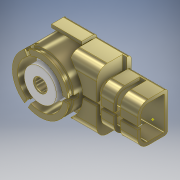
# Autodesk Inventor part: U.FL_Female
Saved by Autodesk Inventor 2018 (Build 220112000, 112)
## iProperties
Created: 2018-07-13
Part Number: U.FL_Female
Material: Copper
Document SubType Name: Modeling
Designer: Bradley
Density: 8.94 g/cm^3
Appearance: Gold - Metal
Author: Bradley
Autodesk Inventor part; units mm, degrees
ref_plane "YZ Plane" through (0, 0, 0) normal (1, 0, 0) x (0, 1, 0)
ref_plane "XZ Plane" through (0, 0, 0) normal (0, 1, 0) x (-1, 0, 0)
ref_plane "XY Plane" through (0, 0, 0) normal (0, 0, 1) x (1, 0, 0)
sketch "Sketch1" plane through (0, 0, 0) normal (0, 0, 1) x (1, 0, 0)
  line L0 (0, 0.565) -> (0, -0.565)
  line L1 (0, -0.565) -> (0.275, -0.565)
  line L2 (0.275, -0.565) -> (0.275, -1.365)
  line L3 (0.275, -1.365) -> (0.75, -1.365)
  line L4 (0.75, -1.365) -> (0.75, -0.495)
  line L5 (0.75, -0.495) -> (1.05, -0.495)
  line L6 (1.05, -0.495) -> (1.05, -1.365)
  line L7 (1.05, -1.365) -> (1.3, -1.365)
  line L8 (1.3, -1.365) -> (1.3, -1.295)
  line L9 (1.3, -1.295) -> (1.2, -1.295)
  line L10 (1.2, -1.295) -> (1.2, -1.095)
  line L11 (1.2, -1.095) -> (1.3, -1.095)
  line L12 (1.3, -1.095) -> (1.3, 0.565)
  line L13 (1.3, 0.565) -> (0, 0.565)
  point P0 (0, 0)
  point P1 (0, 0)
  dimension "d0" = 2.6
  dimension "d1" = 1.93
  dimension "d2" = 2.1
  dimension "d3" = 1.5
  dimension "d4" = 0.55
  dimension "d5" = 0.8
  dimension "d6" = 0.07
  dimension "d7" = 0.6
  dimension "d8" = 0.2
  dimension "d9" = 0.1
  constraints: 28 end point, 10 perpendicular, 4 point on line, 1 coincident, 1 midpoint, 1 vertical
  measures "d0" diameter of L12 L0
  measures "d1" distance between parallel lines of L7 L13
  measures "d2" diameter of L6 L0
  measures "d3" diameter of L4 L0
  measures "d4" diameter of L2 L0
  measures "d5" distance of L1.end L2.end
  measures "d6" distance between parallel lines of L5 L1
  measures "d7" distance between parallel lines of L11 L5
  measures "d8" distance of L9.end L10.end
  measures "d9" distance of L10.end L11.end
revolve "Revolution1" add sketch "Sketch1" angle 360 about axis through (0, 0.565, 0) along (0, -1, 0)
sketch "Sketch2" plane through (0, 0.565, 0) normal (0, 1, 0) x (1, 0, 0)
  circle A0 centre (0, 0) radius 1.3 projected
  line L0 (-0.7, -1.5) -> (0.7, -1.5)
  line L1 (0.7, -1.5) -> (0.7, 1.5)
  line L2 (0.7, 1.5) -> (-0.7, 1.5)
  line L3 (-0.7, 1.5) -> (-0.7, -1.5)
  line L4 (0.7, -1.25) -> (0.8, -1.25)
  line L5 (0.8, -1.25) -> (0.8, 1.25)
  line L6 (0.8, 1.25) -> (0.7, 1.25)
  line L7 (0.7, 1.25) -> (0.7, -1.25)
  point P0 (0, 0)
  point P1 (0, -1.5)
  point P2 (-0.7, 0)
  point P3 (0.7, 0)
  dimension "d11" = 1.4
  dimension "d12" = 3
  dimension "d13" = 2.5
  dimension "d14" = 0.1
  constraints: 16 end point, 4 midpoint, 4 parallel, 2 horizontal, 2 perpendicular, 1 horizontal alignment, 1 point on line, 1 vertical alignment
  measures "d11" distance of L0.start L0.end
  measures "d12" distance of L2.end L0.start
  measures "d13" distance of L4.end L5.end
  measures "d14" distance of L4.start L4.end
extrude "Extrusion1" add sketch "Sketch2" against normal blind 0.7 contours L5 A0 L1 | A0 L1 L6 L5 | L5 L4 L1 A0 | L1 A0 L3 | A0 L3 L2 L1 | L1 L0 L3 A0
sketch "Sketch3" plane through (-0.7, 0.565, -1.5) normal (0, 1, 0) x (1, 0, 0)
  arc A0 (1.5, -2.5247) -> (1.5, -0.4753) centre (0.7, -1.5) ccw projected
  line L0 (1.5, -0.4753) -> (1.5, -0.25) projected
  line L1 (1.5, -0.25) -> (1.4, -0.25) projected
  line L2 (1.4, -0.25) -> (1.4, 0) projected
  line L3 (1.4, 0) -> (0, 0) projected
  line L4 (0, 0) -> (0, -0.4046) projected
  arc A1 (0, -0.4046) -> (0, -2.5954) centre (0.7, -1.5) ccw projected
  line L5 (0, -2.5954) -> (0, -3) projected
  line L6 (0, -3) -> (1.4, -3) projected
  line L7 (1.4, -3) -> (1.4, -2.75) projected
  line L8 (1.4, -2.75) -> (1.5, -2.75) projected
  line L9 (1.5, -2.75) -> (1.5, -2.5247) projected
  line L10 (1.5, -0.075) -> (3, -0.075)
  line L11 (3, -0.075) -> (3, -2.925)
  line L12 (3, -2.925) -> (1.5, -2.925)
  line L13 (1.5, -2.925) -> (1.5, -0.075)
  line L14 (3, -0.575) -> (4.7, -0.575)
  line L15 (4.7, -0.575) -> (4.7, -2.425)
  line L16 (4.7, -2.425) -> (3, -2.425)
  line L17 (3, -2.425) -> (3, -0.575)
  arc A2 (1.5, -2.5247) -> (1.5, -0.4753) centre (0.7, -1.5) ccw
  arc A3 (1.5, -2.5247) -> (1.5, -0.4753) centre (0.7, -1.5) ccw projected
  point P0 (0.7, -1.5)
  point P1 (1.5, -1.5)
  point P2 (3, -1.5)
  dimension "d17" = 2.85
  dimension "d18" = 1.5
  dimension "d19" = 1.85
  dimension "d20" = 4
  constraints: 16 end point, 4 parallel, 4 point on circle, 3 midpoint, 3 point on line, 2 horizontal, 2 perpendicular, 1 centre point, 1 collinear, 1 concentric, 1 horizontal alignment
  measures "d17" distance of L10.end L11.end
  measures "d18" distance of L10.start L10.end
  measures "d19" distance of L14.end L15.end
  measures "d20" distance from line of L15 point (0.7, -1.5)
extrude "Extrusion2" add sketch "Sketch3" against normal blind 1.4 contours A0 L0 L13 L10 L11 L12 L9 | L11 L14 L15 L16
sketch "Sketch4" plane through (0, -1.365, 0) normal (0, -1, 0) x (1, 0, 0)
  circle A0 centre (0, 0) radius 1.3 projected
  circle A1 centre (0, 0) radius 1.05 projected
  circle A2 centre (0, 0) radius 1.05 projected
  arc A3 (1.0452, -0.1) -> (1.0452, 0.1) centre (0, 0) ccw
  circle A4 centre (0, 0) radius 1.3 projected
  arc A5 (1.2961, -0.1) -> (1.2961, 0.1) centre (0, 0) ccw
  line L0 (1.0452, 0.1) -> (1.2961, 0.1)
  line L1 (1.2961, -0.1) -> (1.0452, -0.1)
  circle A6 centre (0, 0) radius 1.05 projected
  arc A7 (-0.436, 0.9552) -> (-0.6092, 0.8552) centre (0, 0) ccw
  arc A8 (-0.5615, 1.1725) -> (-0.7347, 1.0725) centre (0, 0) ccw
  line L2 (-0.6092, 0.8552) -> (-0.7347, 1.0725)
  line L3 (-0.5615, 1.1725) -> (-0.436, 0.9552)
  arc A9 (-0.6092, -0.8552) -> (-0.436, -0.9552) centre (0, 0) ccw
  arc A10 (-0.7347, -1.0725) -> (-0.5615, -1.1725) centre (0, 0) ccw
  line L4 (-0.436, -0.9552) -> (-0.5615, -1.1725)
  line L5 (-0.7347, -1.0725) -> (-0.6092, -0.8552)
  point P0 (0, 0)
  dimension "d23" = 0.2
  dimension "d26" = 360
  constraints: 16 point on circle, 12 end point, 6 centre point, 2 concentric, 2 horizontal, 1 parallel, 31 other
  measures "d23" distance between parallel lines of L1 L0
extrude "Extrusion3" cut sketch "Sketch4" against normal blind 0.5 contours A0 L1 A1 L0 | L3 A1 L2 A0 | A0 L5 A1 L4
fillet "Fillet1" radius 0.5 4 edges at (1.55, -0.835, 1.425) (3.15, -0.835, 0.925) (1.55, -0.835, -1.425) (3.15, -0.835, -0.925)
sketch "Sketch5" plane through (1.0452, -1.365, -0.1) normal (0, -1, 0) x (1, 0, 0)
  arc A0 (-1.7452, -0.9954) -> (-0.2452, -0.9247) centre (-1.0452, 0.1) ccw projected
  line L0 (-1.7452, -0.9954) -> (-1.7452, -1.4) projected
  line L1 (-1.7452, -1.4) -> (-0.3452, -1.4) projected
  line L2 (-0.3452, -1.4) -> (-0.3452, -1.15) projected
  line L3 (-0.3452, -1.15) -> (-0.2452, -1.15) projected
  line L4 (-0.2452, -1.15) -> (-0.2452, -0.9247) projected
  arc A1 (-0.2452, 1.1247) -> (-1.7452, 1.1954) centre (-1.0452, 0.1) ccw projected
  line L5 (-0.2452, 1.1247) -> (-0.2452, 1.35) projected
  line L6 (-0.2452, 1.35) -> (-0.3452, 1.35) projected
  line L7 (-0.3452, 1.35) -> (-0.3452, 1.6) projected
  line L8 (-0.3452, 1.6) -> (-1.7452, 1.6) projected
  line L9 (-1.7452, 1.6) -> (-1.7452, 1.1954) projected
  line L10 (-1.7452, -0.9954) -> (-1.7452, -1.4) projected
  line L11 (-1.7452, -1.25) -> (-0.3452, -1.25)
  line L12 (-1.7452, 1.1954) -> (-1.7452, 1.6) projected
  line L13 (-1.7452, 1.45) -> (-0.3452, 1.45)
  line L14 (-0.3452, 1.6) -> (-0.3452, 1.35) projected
  line L15 (-0.2452, -0.9247) -> (-0.2452, -1.325) projected
  line L16 (-0.2452, -1.325) -> (1.2548, -1.325) projected
  line L17 (1.2548, -1.325) -> (1.2548, -0.825) projected
  line L18 (1.2548, -0.825) -> (-0.1318, -0.825) projected
  line L19 (2.9548, -0.325) -> (1.2548, -0.325) projected
  line L20 (2.9548, -0.325) -> (2.9548, 0.525) projected
  line L21 (1.2548, 0.525) -> (2.9548, 0.525) projected
  line L22 (1.2548, 1.025) -> (1.2548, 0.525) projected
  line L23 (-0.1318, 1.025) -> (1.2548, 1.025) projected
  arc A2 (-0.1318, -0.825) -> (-0.1318, 1.025) centre (-1.0452, 0.1) ccw projected
  line L24 (1.2548, -0.825) -> (-0.1318, -0.825) projected
  line L25 (1.2548, -0.325) -> (1.2548, -0.825) projected
  line L26 (-0.2452, 1.525) -> (-0.2452, 1.1247) projected
  line L27 (-0.1318, 1.025) -> (1.2548, 1.025) projected
  line L28 (1.2548, 1.025) -> (1.2548, 1.525) projected
  line L29 (1.2548, 1.525) -> (-0.2452, 1.525) projected
  line L30 (-0.2452, -1.15) -> (-0.2452, -0.9247) projected
  line L31 (-0.2452, 1.1247) -> (-0.2452, 1.525) projected
  arc A3 (-0.2452, -1.1093) -> (-0.2452, 1.3093) centre (-1.0452, 0.1) ccw
  line L32 (-0.2452, -1.1093) -> (-0.2452, -0.9247)
  line L33 (-0.2452, 1.1247) -> (-0.2452, 1.3093)
  arc A4 (-0.2452, -0.9247) -> (-0.2452, 1.1247) centre (-1.0452, 0.1) ccw
  dimension "d31" = 0.15
  dimension "d32" = 0.15
  dimension "d33" = 0.15
  constraints: 8 end point, 6 point on line, 4 point on circle, 2 centre point, 2 collinear, 1 coincident, 1 parallel, 1 perpendicular, 3 other
  measures "d31" distance between parallel lines of L1 L11
  measures "d32" distance between parallel lines of L8 L13
  measures "d33" radial gap between concentric circles of A3 A2
extrude "Extrusion4" cut sketch "Sketch5" against normal blind 1.75 contours A0 L4 L3 L2 L11 L0 | A4 L18 A3 L4 | A2 L23 A3 L18 | A4 L5 A3 L23 | A1 L9 L13 L7 L6 L5
sketch "Sketch6" plane through (-0.7, -0.835, -1.5) normal (0, -1, 0) x (1, 0, 0)
  line L0 (4.7, 0.575) -> (4.7, 1.075) projected
  line L1 (4.7, 1.075) -> (3, 1.075) projected
  line L2 (3, 1.075) -> (3, 0.575) projected
  line L3 (3, 0.575) -> (4.7, 0.575) projected
  line L4 (3, 1.925) -> (3, 2.425) projected
  line L5 (3, 1.925) -> (4.7, 1.925) projected
  line L6 (4.7, 1.925) -> (4.7, 2.425) projected
  line L7 (4.7, 2.425) -> (3, 2.425) projected
  line L8 (4.7, 2.425) -> (3, 2.425) projected
  line L9 (3.6, 0.575) -> (3.9, 0.575)
  line L10 (3.9, 0.575) -> (3.9, 2.425)
  line L11 (3.9, 2.425) -> (3.6, 2.425)
  line L12 (3.6, 2.425) -> (3.6, 0.575)
  arc A0 (1.8166, 0.575) -> (1.8166, 2.425) centre (0.7, 1.5) ccw projected
  line L13 (3, 0.575) -> (1.8166, 0.575) projected
  line L14 (3, 1.075) -> (3, 0.575) projected
  line L15 (4.7, 1.075) -> (3, 1.075) projected
  line L16 (4.7, 1.075) -> (4.7, 1.925) projected
  line L17 (3, 1.925) -> (4.7, 1.925) projected
  line L18 (3, 2.425) -> (3, 1.925) projected
  line L19 (1.8166, 2.425) -> (3, 2.425) projected
  arc A1 (1.8166, 0.575) -> (1.8166, 2.425) centre (0.7, 1.5) ccw projected
  line L20 (2.1481, 1.425) -> (4.7, 1.425)
  line L21 (4.7, 2.425) -> (4.7, 0.575) projected
  line L22 (4.7, 1.575) -> (2.1481, 1.575)
  line L23 (4.7, 1.425) -> (4.7, 1.575)
  arc A2 (2.1481, 1.425) -> (2.1481, 1.575) centre (0.7, 1.5) ccw
  line L24 (1.5, 0.2907) -> (1.5, 0.075) projected
  line L25 (1.5, 0.075) -> (3, 0.075) projected
  line L26 (3, 0.075) -> (3, 0.575) projected
  line L27 (3, 0.575) -> (1.8166, 0.575) projected
  line L28 (1.8166, 2.425) -> (3, 2.425) projected
  line L29 (3, 2.425) -> (3, 2.925) projected
  line L30 (3, 2.925) -> (1.5, 2.925) projected
  line L31 (1.5, 2.925) -> (1.5, 2.7093) projected
  line L32 (3, 0.575) -> (3, 0.075) projected
  line L33 (3, 0.075) -> (2.8, 0.075)
  line L34 (2.8, 0.075) -> (2.8, 2.925)
  line L35 (2.8, 2.925) -> (3, 2.925)
  line L36 (3, 2.925) -> (3, 0.075)
  point P0 (0.7, 1.5)
  dimension "d36" = 0.8
  dimension "d37" = 0.3
  dimension "d40" = 0.15
  dimension "d48" = 0.2
  constraints: 22 end point, 7 point on line, 6 parallel, 4 point on circle, 3 perpendicular, 2 horizontal, 1 centre point, 1 collinear, 1 concentric, 2 other
  measures "d36" distance between parallel lines of L0 L10
  measures "d37" distance between parallel lines of L10 L12
  measures "d40" distance between parallel lines of L22 L20
  measures "d48" distance between parallel lines of L36 L34
extrude "Extrusion6" cut sketch "Sketch6" against normal blind 1.2 contours L3 L12 L1 L10 | L1 L12 L20 L10 | L20 L10 L22 L16 | L20 L12 L22 L10 | L13 L34 L20 L36 L2 | L26 L25 L34 L13 | L20 L36 L22 L12 | L22 L12 L5 L10 | L20 L34 L22 L36 | L5 L12 L7 L10 | L20 A0 L22 L34 | L22 L34 L19 L4 L36 | L34 L30 L29 L19
sketch "Sketch7" plane through (4, 0.565, 0.925) normal (1, 0, 0) x (0, 0, -1)
  line L0 (1, -0.2) -> (1, -1.4) projected
  line L1 (1.35, -1.4) -> (1, -1.4) projected
  arc A0 (1.35, -1.4) -> (1.85, -0.9) centre (1.35, -0.9) ccw projected
  line L2 (1.85, 0) -> (1.85, -0.9) projected
  line L3 (0, 0) -> (1.85, 0) projected
  line L4 (0, 0) -> (0, -0.9) projected
  arc A1 (0, -0.9) -> (0.5, -1.4) centre (0.5, -0.9) ccw projected
  line L5 (0.85, -1.4) -> (0.5, -1.4) projected
  line L6 (0.85, -1.4) -> (0.85, -0.2) projected
  line L7 (0.85, -0.2) -> (1, -0.2) projected
  arc A2 (1.35, -1.25) -> (1.7, -0.9) centre (1.35, -0.9) ccw
  line L8 (1.35, -1.25) -> (0.5, -1.25)
  arc A3 (0.15, -0.9) -> (0.5, -1.25) centre (0.5, -0.9) ccw
  line L9 (0.15, -0.9) -> (0.15, -0.15)
  line L10 (0.15, -0.15) -> (1.7, -0.15)
  line L11 (1.7, -0.15) -> (1.7, -0.9)
  point P0 (0.925, -0.565)
  dimension "d43" = 0.15
  constraints: 8 end point, 4 point on circle, 2 centre point, 1 perpendicular, 1 tangent, 4 other
  measures "d43" radial gap between concentric circles of A0 A2
extrude "Extrusion7" cut sketch "Sketch7" against normal up to surface contours L7 L6 L8 A3 L9 L10 L11 A2 L0 | L0 L8 L6 L7 round surface about axis through (0, -0.265, 0) along (0, -1, 0) radius 1.3 far side no
sketch "Sketch8" plane through (-0.7, 0.565, -1.5) normal (0, 1, 0) x (1, 0, 0)
  line L0 (1.5, -0.25) -> (1.4, -0.25) projected
  line L1 (1.4, -0.25) -> (1.4, 0) projected
  line L2 (1.4, 0) -> (0, 0) projected
  line L3 (0, 0) -> (0, -0.4046) projected
  arc A0 (0, -0.4046) -> (0, -2.5954) centre (0.7, -1.5) ccw projected
  line L4 (0, -2.5954) -> (0, -3) projected
  line L5 (0, -3) -> (1.4, -3) projected
  line L6 (1.4, -3) -> (1.4, -2.75) projected
  line L7 (1.4, -2.75) -> (1.5, -2.75) projected
  line L8 (1.5, -2.75) -> (1.5, -2.925) projected
  line L9 (1.5, -2.925) -> (3, -2.925) projected
  line L10 (3, -2.925) -> (3, -2.425) projected
  line L11 (3, -2.425) -> (4.7, -2.425) projected
  line L12 (4.7, -2.425) -> (4.7, -0.575) projected
  line L13 (4.7, -0.575) -> (3, -0.575) projected
  line L14 (3, -0.575) -> (3, -0.075) projected
  line L15 (3, -0.075) -> (1.5, -0.075) projected
  line L16 (1.5, -0.075) -> (1.5, -0.25) projected
  arc A1 (0, -0.4046) -> (0, -2.5954) centre (0.7, -1.5) ccw projected
  line L17 (0, -2.5954) -> (0, -1.9)
  line L18 (0, -1.9) -> (-0.5369, -1.9)
  line L19 (-0.5369, -1.1) -> (0, -1.1)
  line L20 (0, -1.1) -> (0, -0.4046)
  line L21 (0, -1.1) -> (0, -1.9) construction
  point P0 (0.7, -1.5)
  point P1 (0, -1.5)
  dimension "d49" = 0.8
  constraints: 10 end point, 2 point on circle, 2 vertical, 1 horizontal, 1 horizontal alignment, 1 midpoint, 1 parallel, 1 perpendicular
  measures "d49" distance between parallel lines of L18 L19
extrude "Extrusion8" cut sketch "Sketch8" against normal blind 0.3 contours L20 L19 A0 | L18 L17 A0
sketch "Sketch9" plane through (-0.7, 0.265, -1.5) normal (0, 1, 0) x (1, 0, 0)
  arc A0 (0, -0.4046) -> (-0.5369, -1.1) centre (0.7, -1.5) ccw projected
  line L0 (0, -1.1) -> (-0.5369, -1.1) projected
  line L1 (0, -0.4046) -> (0, -1.1) projected
  line L2 (0, -1.9) -> (0, -2.5954) projected
  line L3 (-0.5369, -1.9) -> (0, -1.9) projected
  arc A1 (-0.5369, -1.9) -> (0, -2.5954) centre (0.7, -1.5) ccw projected
  line L4 (0, -0.4046) -> (0, -1.1) projected
  line L5 (0, -1.1) -> (-0.5369, -1.1) projected
  arc A2 (0, -0.6515) -> (-0.3247, -1.1) centre (0.7, -1.5) ccw
  line L6 (-0.5369, -1.9) -> (0, -1.9) projected
  line L7 (0, -1.9) -> (0, -3) projected
  arc A3 (-0.3247, -1.9) -> (0, -2.3485) centre (0.7, -1.5) ccw
  arc A4 (0, -0.4046) -> (-0.5369, -1.1) centre (0.7, -1.5) ccw projected
  point P0 (0.7, -1.5)
  dimension "d52" = 0.2
  constraints: 4 point on circle, 4 point on line, 3 concentric, 2 centre point
  measures "d52" radial gap between concentric circles of A0 A2
extrude "Extrusion9" cut sketch "Sketch9" against normal blind 0.3 contours L1 L0 A2 | L2 A3 L3
fillet "Fillet2" radius 0.15 10 edges at (0, 0.565, 1.5) (1.55, 0.565, 1.425) (3.15, 0.565, 0.925) (3.15, 0.565, -0.925) (1.55, 0.565, -1.425) (0, 0.565, -1.5) (-0.7, 0.415, 0.4) (-0.7, 0.115, 0.4) (-0.7, 0.415, -0.4) (-0.7, 0.115, -0.4)
fillet "Fillet2" radius 0.05 5 edges at (0, 0.385, 1.35) (0, 0.385, -1.35) (2.5219, 0.415, 0.775) (2.5219, 0.415, -0.775) (-0.275, -1.365, 0)
fillet "Fillet2" radius 0.3 1 edges at (-1.3, 0.565, 0)
sketch "Sketch10" plane through (4, 0.565, 0.775) normal (0, 1, 0) x (1, 0, 0)
  arc A0 (-4.9165, 1.175) -> (-4.9165, 0.375) centre (-4, 0.775) ccw projected
  line L0 (-4.9165, 0.375) -> (-4.85, 0.375) projected
  arc A1 (-4.7, 0.225) -> (-4.85, 0.375) centre (-4.85, 0.225) ccw projected
  line L1 (-4.7, 0.225) -> (-4.7, -0.575) projected
  line L2 (-3.3, -0.575) -> (-4.7, -0.575) projected
  line L3 (-3.3, -0.575) -> (-3.3, -0.475) projected
  line L4 (-3.3, -0.475) -> (-3.2, -0.475) projected
  line L5 (-3.2, -0.475) -> (-3.2, -0.5) projected
  line L6 (-1.7, -0.5) -> (-3.2, -0.5) projected
  line L7 (-1.7, -0.5) -> (-1.7, 0) projected
  line L8 (0, 0) -> (-1.7, 0) projected
  line L9 (0, 0) -> (0, 1.55) projected
  line L10 (-1.7, 1.55) -> (0, 1.55) projected
  line L11 (-1.7, 1.55) -> (-1.7, 2.05) projected
  line L12 (-3.2, 2.05) -> (-1.7, 2.05) projected
  line L13 (-3.2, 2.05) -> (-3.2, 2.025) projected
  line L14 (-3.2, 2.025) -> (-3.3, 2.025) projected
  line L15 (-3.3, 2.025) -> (-3.3, 2.125) projected
  line L16 (-4.7, 2.125) -> (-3.3, 2.125) projected
  line L17 (-4.7, 2.125) -> (-4.7, 1.325) projected
  arc A2 (-4.85, 1.175) -> (-4.7, 1.325) centre (-4.85, 1.325) ccw projected
  line L18 (-4.85, 1.175) -> (-4.9165, 1.175) projected
  line L19 (-4.15, 0.025) -> (-3.85, 0.025)
  line L20 (-3.85, 0.025) -> (-3.85, 1.525)
  line L21 (-3.85, 1.525) -> (-4.15, 1.525)
  line L22 (-4.15, 1.525) -> (-4.15, 0.025)
  line L23 (-2.1, 0.525) -> (-1.3, 0.525)
  line L24 (-1.3, 0.525) -> (-1.3, 1.025)
  line L25 (-1.3, 1.025) -> (-2.1, 1.025)
  line L26 (-2.1, 1.025) -> (-2.1, 0.525)
  line L27 (-0.45, 0.275) -> (-0.25, 0.275)
  line L28 (-0.25, 0.275) -> (-0.25, 1.275)
  line L29 (-0.25, 1.275) -> (-0.45, 1.275)
  line L30 (-0.45, 1.275) -> (-0.45, 0.275)
  point P0 (-4.15, 0.775)
  point P1 (-2.1, 0.775)
  point P2 (-0.45, 0.775)
  point P3 (-4, 0.025)
  point P4 (-1.7, 1.025)
  dimension "d56" = 1.5
  dimension "d57" = 0.3
  dimension "d58" = 0.5
  dimension "d59" = 0.8
  dimension "d60" = 1
  dimension "d61" = 0.2
  dimension "d62" = 0.25
  constraints: 24 end point, 6 parallel, 5 midpoint, 3 horizontal, 3 horizontal alignment, 3 perpendicular, 2 vertical alignment
  measures "d56" distance of L21.end L19.start
  measures "d57" distance of L19.start L19.end
  measures "d58" distance of L25.end L23.start
  measures "d59" distance of L24.end L25.end
  measures "d60" distance of L29.end L27.start
  measures "d61" distance of L27.start L27.end
  measures "d62" distance between parallel lines of L9 L28
extrude "Extrusion10" cut sketch "Sketch10" against normal blind 0.05 contours L22 L21 L20 L19 | L26 L25 L24 L23 | L30 L29 L28 L27
fillet "Fillet3" radius 0.024 36 edges at (2.7, 0.54, -0.25) (2.7, 0.515, 0) (2.7, 0.54, 0.25) (1.9, 0.54, -0.25) (2.3, 0.515, -0.25) (1.9, 0.54, 0.25) (1.9, 0.515, 0) (2.3, 0.515, 0.25) (3.75, 0.54, -0.5) (3.75, 0.515, 0) (3.75, 0.54, 0.5) (3.55, 0.54, -0.5) (3.65, 0.515, -0.5) (3.55, 0.54, 0.5) (3.55, 0.515, 0) (3.65, 0.515, 0.5) (0.15, 0.54, -0.75) (0.15, 0.515, 0) (0.15, 0.54, 0.75) (-0.15, 0.54, -0.75) (0, 0.515, -0.75) (-0.15, 0.54, 0.75) (-0.15, 0.515, 0) (0, 0.515, 0.75) (-0.15, 0.565, 0) (0, 0.565, 0.75) (0.15, 0.565, 0) (0, 0.565, -0.75) (2.7, 0.565, 0) (2.3, 0.565, 0.25) (1.9, 0.565, 0) (2.3, 0.565, -0.25) (3.55, 0.565, 0) (3.75, 0.565, 0) (3.65, 0.565, 0.5) (3.65, 0.565, -0.5)
sketch "Sketch11" plane through (0, 0, 0) normal (0, 0, 1) x (1, 0, 0)
  line L0 (4, 0.415) -> (1.0791, 0.415) projected
  line L1 (1.0791, 0.415) -> (4, 0.415) projected
  line L2 (1.0791, 0.415) -> (1.0791, 0.415) projected
  line L3 (1.4481, -0.685) -> (2.1, -0.685) projected
  line L4 (1.3863, -0.685) -> (1.4481, -0.685) projected
  line L5 (2.1, -0.685) -> (1.3863, -0.685) projected
  line L6 (3.2, -0.685) -> (4, -0.685) projected
  line L7 (4, -0.685) -> (3.2, -0.685) projected
  line L8 (1.4481, -0.685) -> (2.1, -0.685) construction
  line L9 (1.774, -0.685) -> (1.774, 0.415) construction
  line L10 (1.0791, 0.415) -> (4, 0.415) construction
  line L11 (4, 0.415) -> (4, -0.335) construction
  line L12 (4, -0.685) -> (4, 0.415) construction
  line L13 (2.3, -0.685) -> (2.9, -0.685) projected
  line L14 (2.9, -0.685) -> (2.3, -0.685) construction
  line L15 (2.6, -0.685) -> (2.6, 0.415) construction
  point P0 (0, 0)
  point P1 (1.774, -0.135)
  point P2 (2.6, -0.135)
  point P3 (4, -0.135)
  constraints: 6 end point, 5 midpoint, 2 perpendicular, 2 point on line, 1 collinear
equation "\"d32\" = d31"
equation "\"d33\" = d31"
body "Solid1"
